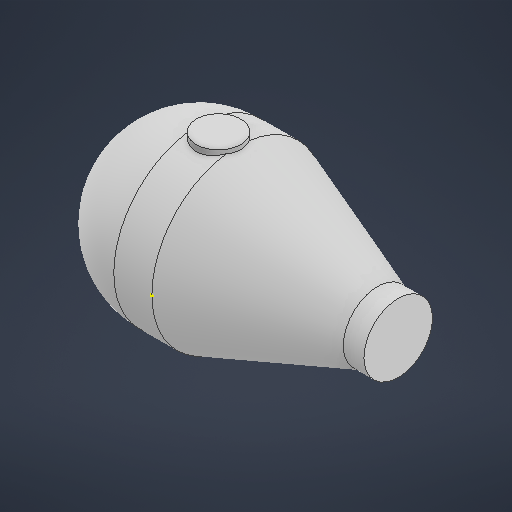
# Autodesk Inventor part: diff
Saved by Autodesk Inventor 2026.1 (Build 301233000, 233)
## iProperties
Created: 2026-07-07
Part Number: diff
Material: Generic
Document SubType Name: Modeling
Designer: tasle
Density: 1.48334 g/cm^3
Appearance: Default
Mass: 23000 g
Surface Area: 3285.73 cm^2
Volume: 15505.6 cm^3
Author: tasle
Autodesk Inventor part; units mm, degrees
ref_plane "YZ Plane" through (0, 0, 0) normal (1, 0, 0) x (0, 1, 0)
ref_plane "XZ Plane" through (0, 0, 0) normal (0, 1, 0) x (-1, 0, 0)
ref_plane "XY Plane" through (0, 0, 0) normal (0, 0, 1) x (1, 0, 0)
sketch "Sketch1" plane through (0, 0, 0) normal (0, 1, 0) x (-1, 0, 0)
  line L0 (0, 0) -> (60, 0)
  line L1 (60, 0) -> (60, -270)
  line L2 (60, -270) -> (0, -270)
  line L3 (0, -270) -> (0, 0)
  line L4 (-220, -81.3644) -> (-252.5016, -81.3644)
  line L5 (-252.5016, -81.3644) -> (-252.5016, -189.3697)
  line L6 (-252.5016, -189.3697) -> (-220, -189.3697)
  line L7 (-220, -189.3697) -> (-220, -81.3644)
  line L8 (0, -135) -> (-220, -135)
  line L9 (-220, -189.3697) -> (0, -270)
  arc A0 (60, -270) -> (60, 0) centre (60, -135) ccw
  line L10 (0, 0) -> (-220, -81.3644)
  line L11 (-252.5016, -135.3671) -> (195, -135)
  point P0 (-220, -135.3404)
  point P1 (0, -135.16)
  dimension "d0" = 270
  dimension "d1" = 60
  dimension "d2" = 220
  constraints: 24 end point, 4 parallel, 3 horizontal, 3 midpoint, 3 point on circle, 2 perpendicular, 1 centre point, 1 point on line
  measures "d0" distance of L0.end L1.end
  measures "d1" distance of L1.end L2.end
  measures "d2" distance of L8.start L8.end
revolve "Revolution1" add sketch "Sketch1" angle 360 about axis through (252.5016, 0, -135.3671) along (-0.9999997, 0, 0.0008203) picked at (65.4242, -45.365) contours L0 L1 L11 L3 | L3 L8 L7 L10 | A0 L11 L1 | L7 L11 L5 L4
sketch "Sketch2" plane through (0, 0, 0) normal (0, 1, 0) x (-1, 0, 0)
  point P0 (0, 0)
sketch "Sketch3" plane through (0, 0, 0) normal (0, 1, 0) x (-1, 0, 0)
  circle A0 centre (30.1107, -134.9753) radius 35
  line L0 (0.2217, -270.3197) -> (0, 0) projected
  dimension "d4" = 70
  dimension "d5" = 30
  constraints: 1 centre point
  measures "d4" diameter of A0
  measures "d5" distance from line of L0 A0.centre
extrude "Extrusion1" add sketch "Sketch3" along normal mid plane 280
body "Solid1"
